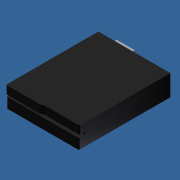
# Autodesk Inventor part: PC
Saved by Autodesk Inventor 2012 (Build 160160000, 160)
## iProperties
Created: 2012-03-08
Part Number: PC
Material: Default
Document SubType Name: Modeling
Designer: esv
Density: 1 g/cm^3
Mass: 13079.6 g
Surface Area: 4401.97 cm^2
Volume: 13079.6 cm^3
Author: esv
Autodesk Inventor part; units mm, degrees
ref_plane "YZ Plane" through (0, 0, 0) normal (1, 0, 0) x (0, 1, 0)
ref_plane "XZ Plane" through (0, 0, 0) normal (0, 1, 0) x (-1, 0, 0)
ref_plane "XY Plane" through (0, 0, 0) normal (0, 0, 1) x (1, 0, 0)
sketch "Sketch1" plane through (0, 0, 0) normal (0, 0, 1) x (1, 0, 0)
  line L0 (0, 0) -> (330.2, 0)
  line L1 (330.2, 0) -> (330.2, 95.25)
  line L2 (330.2, 95.25) -> (0, 95.25)
  line L3 (0, 95.25) -> (0, 0)
  dimension "d0" = 95.25
  dimension "d1" = 330.2
  constraints: 8 end point, 2 parallel, 1 horizontal, 1 perpendicular
  measures "d0" distance of L2.end L0.start
  measures "d1" distance of L0.start L0.end
extrude "Extrusion1" add sketch "Sketch1" along normal blind 390.525
sketch "Sketch2" plane through (0, 95.25, 0) normal (0, 1, 0) x (1, 0, 0)
  line L0 (330.2, 0) -> (330.2, -390.525) projected
  line L1 (0, 0) -> (0, -390.525) projected
  line L2 (172.1995, -415.925) -> (330.2, -415.925)
  line L3 (330.2, -415.925) -> (330.2, -390.525)
  line L4 (152.4, -422.275) -> (0, -422.275)
  line L5 (0, -422.275) -> (0, -390.525)
  line L6 (159.1248, -420.6875) -> (165.4748, -417.5125)
  arc A0 (172.1995, -415.925) -> (165.4748, -417.5125) centre (172.1995, -430.962) ccw
  arc A1 (152.4, -422.275) -> (159.1248, -420.6875) centre (152.4, -407.238) ccw
  line L7 (330.2, -390.525) -> (0, -390.525)
  dimension "d4" = 25.4
  dimension "d6" = 152.4
  dimension "d7" = 6.35
  dimension "d8" = 3.175
  dimension "d9" = 31.75
  dimension "d10" = 158.0005
  constraints: 12 end point, 4 point on circle, 4 tangent, 2 centre point, 2 collinear, 1 equal radius, 1 perpendicular
  measures "d4" distance of L2.end L0.end
  measures "d6" distance of L4.start L4.end
  measures "d7" horizontal distance of L6.start L6.end
  measures "d8" vertical distance of L6.start L6.end
  measures "d9" distance between parallel lines of L7 L4
  measures "d10" distance of L2.start L2.end
extrude "Extrusion2" add sketch "Sketch2" against normal blind 37.084
sketch "Sketch3" plane through (0, 0, 0) normal (0, -1, 0) x (1, 0, 0)
  line L0 (330.2, 0) -> (330.2, 390.525) projected
  line L1 (0, 390.525) -> (330.2, 390.525)
  line L2 (330.2, 390.525) -> (330.2, 419.1)
  line L3 (330.2, 419.1) -> (0, 419.1)
  line L4 (0, 419.1) -> (0, 390.525)
  dimension "d13" = 28.575
  constraints: 8 end point, 2 parallel, 1 collinear, 1 horizontal, 1 perpendicular
  measures "d13" distance between parallel lines of L1 L3
extrude "Extrusion3" add sketch "Sketch3" against normal blind 46.99
fillet "Fillet1" radius 4.318 4 edges at (330.2, 76.708, 415.925) (0, 76.708, 422.275) (0, 23.495, 419.1) (330.2, 23.495, 419.1)
sketch "Sketch4" plane through (0, 0, 0) normal (0, 0, -1) x (-1, 0, 0)
  line L0 (0, 95.25) -> (0, 0) projected
  line L1 (-330.2, 95.25) -> (0, 95.25) projected
  line L2 (-152.0825, 88.9) -> (-68.2625, 88.9)
  line L3 (-68.2625, 88.9) -> (-68.2625, 85.09)
  line L4 (-68.2625, 85.09) -> (-152.0825, 85.09)
  line L5 (-152.0825, 85.09) -> (-152.0825, 88.9)
  dimension "d17" = 68.2625
  dimension "d18" = 6.35
  dimension "d19" = 83.82
  dimension "d20" = 3.81
  constraints: 8 end point, 2 parallel, 1 horizontal, 1 perpendicular
  measures "d17" distance between parallel lines of L0 L3
  measures "d18" distance between parallel lines of L1 L2
  measures "d19" distance of L2.start L2.end
  measures "d20" distance between parallel lines of L2 L4
extrude "Extrusion4" add sketch "Sketch4" along normal blind 15.875
body "Solid1"
